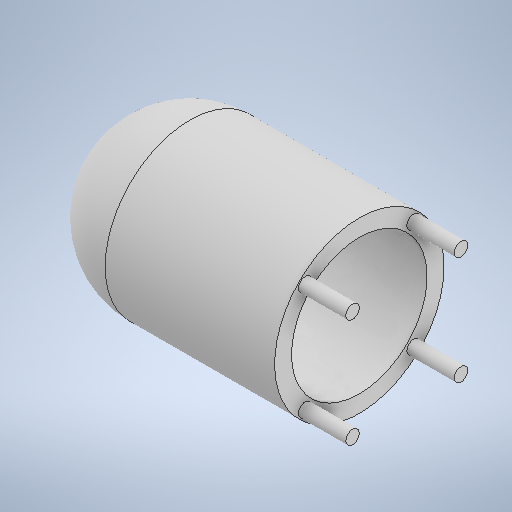
# Autodesk Inventor part: Plasmid Half 1
Saved by Autodesk Inventor 2025 (Build 290162000, 162)
## iProperties
Created: 2024-08-12
Part Number: Plasmid Half 1
Material: Generic
Document SubType Name: Modeling
Designer: kellst1
Density: 1 g/cm^3
Appearance: Default
Author: kellst1
Autodesk Inventor part; units mm, degrees
ref_plane "YZ Plane" through (0, 0, 0) normal (1, 0, 0) x (0, 1, 0)
ref_plane "XZ Plane" through (0, 0, 0) normal (0, 1, 0) x (-1, 0, 0)
ref_plane "XY Plane" through (0, 0, 0) normal (0, 0, 1) x (1, 0, 0)
sketch "Sketch2" plane through (0, 0, 0) normal (1, 0, 0) x (0, 1, 0)
  circle A0 centre (0, 0) radius 10
  circle A1 centre (0, 0) radius 12.5
  dimension "d3" = 20
  dimension "d4" = 25
  constraints: 2 centre point, 2 coincident
  measures "d3" diameter of A0
  measures "d4" diameter of A1
extrude "Extrusion1" add sketch "Sketch2" along normal blind 25
sketch "Sketch3" plane through (0, 0, 0) normal (-1, 0, 0) x (0, 0, 1)
  circle A0 centre (0, 0) radius 10 projected
  arc A1 (10, 0) -> (-10, 0) centre (0, 0) ccw
  circle A2 centre (0, 0) radius 12.5 projected
  arc A3 (12.5, 0) -> (-12.5, 0) centre (0, 0) ccw
  line L0 (-12.5, 0) -> (-10, 0)
  line L1 (10, 0) -> (12.5, 0)
  constraints: 8 point on circle, 4 end point, 2 centre point, 1 collinear, 1 horizontal
revolve "Revolution1" add sketch "Sketch3" angle 180 about axis through (0, 0, 10) along (0, 0, 1) picked at (-11.4487, 1.7949) contours A0 L0 A2 L1
sketch "Sketch5" plane through (25, 0, 0) normal (1, 0, 0) x (0, 0, -1)
  circle A0 centre (-8, 8) radius 1
  point P0 (0, 0)
  dimension "d9" = 2
  constraints: 1 centre point
  measures "d9" diameter of A0
extrude "Extrusion2" add sketch "Sketch5" along normal blind 7
mirror "Mirror1" about plane through (0, 0, 0) normal (0, 0, 1) of "Extrusion2"
mirror "Mirror2" about plane through (0, 0, 0) normal (0, 1, 0) of "Extrusion2", "Mirror1"
body "Solid1"
